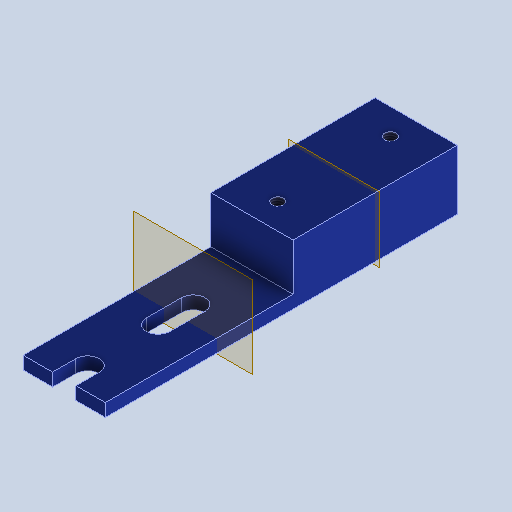
# Autodesk Inventor part: Adapterplatte_Vibrationsdaempfer
Saved by Autodesk Inventor 2025.2 (Build 292293000, 293)
## iProperties
Created: 2025-06-22
Part Number: Adapterplatte_Vibrationsdaempfer
Material: Generisch
Document SubType Name: Modeling
Designer: Jakob
Density: 1 g/cm^3
Appearance: Vorgabe
Author: Jakob
Autodesk Inventor part; units mm, degrees
ref_plane "YZ Plane" through (0, 0, 0) normal (1, 0, 0) x (0, 1, 0)
ref_plane "XZ Plane" through (0, 0, 0) normal (0, 1, 0) x (-1, 0, 0)
ref_plane "XY Plane" through (0, 0, 0) normal (0, 0, 1) x (1, 0, 0)
sketch "Skizze1" plane through (0, 0, 0) normal (0, 0, 1) x (1, 0, 0)
  line L0 (-17.5, 75) -> (17.5, 75)
  line L1 (17.5, 75) -> (17.5, -75)
  line L2 (17.5, -75) -> (-17.5, -75)
  line L3 (-17.5, -75) -> (-17.5, 75)
  line L4 (-17.5, 75) -> (17.5, -75) construction
  line L5 (17.5, 75) -> (-17.5, -75) construction
  point P0 (0, 0)
  dimension "d0" = 35
  dimension "d1" = 150
  constraints: 12 end point, 2 midpoint, 2 parallel, 1 horizontal, 1 perpendicular
  measures "d0" distance of L0.start L0.end
  measures "d1" distance of L0.end L1.end
extrude "Extrusion1" add sketch "Skizze1" along normal blind 5.5
sketch "Skizze2" plane through (0, 0, 5.5) normal (0, 0, 1) x (1, 0, 0)
  arc A0 (5, -65) -> (-5, -65) centre (0, -65) ccw
  line L0 (-17.5, -75) -> (17.5, -75) projected
  line L1 (-5, -65) -> (-5, -75)
  line L2 (5, -65) -> (5, -75)
  line L3 (5, -75) -> (-5, -75)
  line L4 (0, 105) -> (0, -105) projected
  arc A1 (-5, -35) -> (5, -35) centre (0, -35) ccw
  arc A2 (5, -20) -> (-5, -20) centre (0, -20) ccw
  line L5 (-5, -35) -> (-5, -20)
  line L6 (5, -20) -> (5, -35)
  point P0 (0, 0)
  dimension "d4" = 10
  dimension "d5" = 10
  dimension "d32" = 10
  dimension "d33" = 15
  dimension "d34" = 40
  constraints: 10 end point, 6 point on circle, 4 point on line, 4 tangent, 3 centre point, 2 perpendicular, 1 collinear, 1 equal radius, 1 parallel, 1 vertical
  measures "d4" diameter of A0
  measures "d5" distance from line of L0 A0.centre
  measures "d32" diameter of A1
  measures "d33" distance of A2.centre A1.centre
  measures "d34" distance from line of L0 A1.centre
extrude "Extrusion2" cut sketch "Skizze2" against normal through all
sketch "Skizze3" plane through (0, 0, 5.5) normal (0, 0, 1) x (1, 0, 0)
  line L0 (-17.5, 5) -> (17.5, 5)
  line L1 (17.5, 5) -> (17.5, 75)
  line L2 (17.5, 75) -> (-17.5, 75)
  line L3 (-17.5, 75) -> (-17.5, 5)
  line L4 (-17.5, 5) -> (17.5, 75) construction
  line L5 (17.5, 5) -> (-17.5, 75) construction
  line L6 (-17.5, 75) -> (-17.5, -75) projected
  line L7 (17.5, 75) -> (-17.5, 75) projected
  line L8 (17.5, -75) -> (17.5, 75) projected
  point P0 (0, 40)
  point P1 (-4.35, 75)
  point P2 (-17.5, 40)
  dimension "d8" = 70
  constraints: 12 end point, 3 collinear, 3 midpoint, 2 parallel, 1 horizontal, 1 perpendicular
  measures "d8" distance of L2.end L0.start
extrude "Extrusion3" add sketch "Skizze3" along normal blind 20
ref_plane "Arbeitsebene2" through (-17.5, 40, 5.5) normal (0, -1, 0) x (1, 0, 0)
sketch "Skizze5" plane through (0, 0, 25.5) normal (0, 0, 1) x (1, 0, 0)
  line L0 (24.5, 40) -> (-24.5, 40) projected
  line L1 (0, 105) -> (0, -105) projected
  point P0 (0, 0)
  point P1 (0, 16)
  point P2 (0, 64)
  dimension "d23" = 24
  dimension "d24" = 24
  constraints: 2 point on line
  measures "d23" distance from line of L0 point (0, 16)
  measures "d24" distance from line of L0 point (0, 64)
hole "Bohrung2" at (0, 16, 25.5) at (0, 64, 25.5) direction (0, 0, -1) diameter 4.917 depth 16 tip angle 118 thread size "M6x1" class "6H" standard "ISO Metric profile"
ref_plane "Arbeitsebene3" through (-17.5, -27.5, 0) normal (0, -1, 0) x (1, 0, 0)
